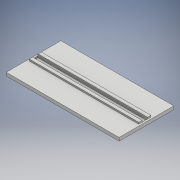
# Autodesk Inventor part: Zijplaat 2
Saved by Autodesk Inventor 2018.3 (Build 223284000, 284)
## iProperties
Created: 2020-11-10
Part Number: Zijplaat 2
Material: Generic
Document SubType Name: Modeling
Designer: daanv
Density: 1 g/cm^3
Appearance: Default
Author: daanv
Autodesk Inventor part; units mm, degrees
ref_plane "YZ Plane" through (0, 0, 0) normal (1, 0, 0) x (0, 1, 0)
ref_plane "XZ Plane" through (0, 0, 0) normal (0, 1, 0) x (-1, 0, 0)
ref_plane "XY Plane" through (0, 0, 0) normal (0, 0, 1) x (1, 0, 0)
sketch "Sketch1" plane through (0, 0, 0) normal (0, 0, 1) x (1, 0, 0)
  line L0 (0, 0) -> (0, 16.7)
  line L1 (0, 16.7) -> (34.5, 16.7)
  line L2 (34.5, 16.7) -> (34.5, 0)
  line L3 (34.5, 0) -> (0, 0)
  dimension "d0" = 16.7
  dimension "d1" = 34.5
  constraints: 8 end point, 3 perpendicular, 1 vertical
  measures "d0" distance of L0.start L0.end
  measures "d1" distance of L0.end L1.end
extrude "Extrusion1" add sketch "Sketch1" along normal blind 1
sketch "Sketch2" plane through (0, 0, 1) normal (0, 0, 1) x (1, 0, 0)
  line L0 (0, 16.7) -> (0, 0) projected
  line L1 (0, 0) -> (34.5, 0) projected
  line L2 (0, 9.2) -> (34.5, 9.2)
  line L3 (34.5, 9.2) -> (34.5, 7.5)
  line L4 (34.5, 7.5) -> (0, 7.5)
  line L5 (0, 7.5) -> (0, 9.2)
  dimension "d4" = 34.5
  dimension "d5" = 1.7
  dimension "d6" = 7.5
  constraints: 8 end point, 3 parallel, 1 horizontal, 1 perpendicular, 1 point on line
  measures "d4" distance of L3.end L4.end
  measures "d5" distance of L2.end L3.end
  measures "d6" distance of L0.start L2.start
extrude "Extrusion2" cut sketch "Sketch2" against normal blind 0.5
sketch "Sketch3" plane through (0, 0, 0.5) normal (0, 0, 1) x (1, 0, 0)
  line L0 (34.5, 7.5) -> (0, 7.5) projected
  line L1 (34.5, 7.5) -> (0, 7.5) projected
  line L2 (0, 9.2) -> (0.5, 9.2)
  line L3 (0.5, 9.2) -> (0.5, 7.5)
  line L4 (0.5, 7.5) -> (0, 7.5)
  line L5 (0, 7.5) -> (0, 9.2)
  line L6 (34.5, 9.2) -> (34, 9.2)
  line L7 (34, 9.2) -> (34, 7.5)
  line L8 (34, 7.5) -> (34.5, 7.5)
  line L9 (34.5, 7.5) -> (34.5, 9.2)
  point P0 (0, 0)
  dimension "d9" = 0.5
  dimension "d10" = 0.5
  constraints: 16 end point, 4 parallel, 2 horizontal, 2 perpendicular, 2 point on line
  measures "d9" distance of L3.end L4.end
  measures "d10" distance of L8.end L7.end
extrude "Extrusion3" add sketch "Sketch3" along normal blind 0.5
sketch "Sketch4" plane through (0, 0, 1) normal (0, 0, 1) x (1, 0, 0)
  line L0 (0.5, 10.2) -> (34, 10.2)
  line L1 (34, 10.2) -> (34, 9.2)
  line L2 (34, 9.2) -> (0.5, 9.2)
  line L3 (0.5, 9.2) -> (0.5, 10.2)
  line L4 (34, 7.5) -> (0.5, 7.5)
  line L5 (0.5, 7.5) -> (0.5, 6.5)
  line L6 (0.5, 6.5) -> (34, 6.5)
  line L7 (34, 6.5) -> (34, 7.5)
  dimension "d13" = 1
  dimension "d14" = 1
  constraints: 16 end point, 4 parallel, 2 horizontal, 2 perpendicular, 1 point on line
  measures "d13" distance of L5.end L4.end
  measures "d14" distance of L2.end L0.start
extrude "Extrusion4" add sketch "Sketch4" along normal blind 0.5
body "Solid1"
